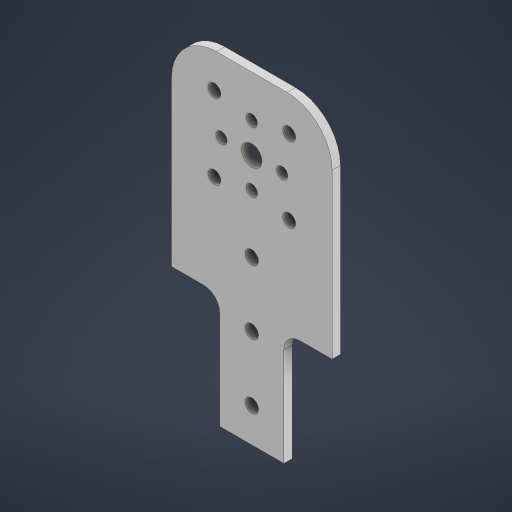
# Autodesk Inventor part: Arm Plate3
Saved by Autodesk Inventor 2024 (Build 280153000, 153)
## iProperties
Created: 2023-10-19
Part Number: Arm Plate3
Material: Generic
Document SubType Name: Modeling
Designer: ellen
Density: 1 g/cm^3
Appearance: Default
Author: ellen
Autodesk Inventor part; units mm, degrees
ref_plane "YZ Plane" through (0, 0, 0) normal (1, 0, 0) x (0, 1, 0)
ref_plane "XZ Plane" through (0, 0, 0) normal (0, 1, 0) x (-1, 0, 0)
ref_plane "XY Plane" through (0, 0, 0) normal (0, 0, 1) x (1, 0, 0)
sketch "Sketch1" plane through (0, 0, 0) normal (0, 0, 1) x (1, 0, 0)
  line L0 (63.5, 76.2) -> (0, 76.2)
  line L1 (0, 76.2) -> (0, 53.975)
  circle A0 centre (31.75, 47.625) radius 4.05
  line L2 (19.05, -6.35) -> (44.45, -6.35)
  line L3 (63.5, 53.975) -> (63.5, 76.2)
  line L4 (31.75, 76.2) -> (31.75, -6.35)
  circle A1 centre (31.75, 12.7) radius 2.6543
  circle A2 centre (31.75, -12.7) radius 2.6543
  circle A3 centre (31.75, -38.1) radius 2.6604
  line L5 (63.5, 53.975) -> (63.5, -6.35)
  line L6 (63.5, -6.35) -> (0, -6.35)
  line L7 (0, -6.35) -> (0, 53.975)
  line L8 (19.05, -6.35) -> (19.05, -51.598)
  line L9 (19.05, -51.598) -> (44.45, -51.598)
  line L10 (44.45, -51.598) -> (44.45, -6.35)
  point P0 (0, 0)
  dimension "d0" = 63.5
  dimension "d2" = 8.1
  dimension "d5" = 28.575
  dimension "d50" = 82.55
  dimension "d54" = 5.3086
  dimension "d55" = 63.5
  dimension "d59" = 25.4
  dimension "d60" = 25.4
  dimension "d61" = 25.4
  constraints: 22 end point, 5 perpendicular, 5 point on line, 4 centre point, 2 midpoint, 2 parallel, 2 vertical, 1 equal radius, 1 horizontal, 1 other
  measures "d0" distance of L0.end L0.start
  measures "d2" diameter of A0
  measures "d5" distance of A0.centre L4.start
  measures "d50" distance between parallel lines of L2 L0
  measures "d54" diameter of A1
  measures "d55" distance from line of L0 A1.centre
  measures "d59" distance of A2.centre A1.centre
  measures "d60" distance of A3.centre A2.centre
  measures "d61" distance of L8.end L9.end
extrude "Extrusion1" add sketch "Sketch1" along normal blind 3.302 contours L3 L5 L6 L2 L4 A1 A0 L0 | L4 A0 A1 L2 L6 L7 L1 L0 | L10 L9 L8 L2
fillet "Fillet11" radius 17.78 1 edges at (63.5, 76.2, 1.651)
fillet "Fillet12" radius 17.78 1 edges at (0, 76.2, 1.651)
sketch "Sketch3" plane through (0, 0, 3.302) normal (0, 0, 1) x (1, 0, 0)
  circle A0 centre (31.75, 47.625) radius 4.05 projected
  circle A1 centre (31.75, 47.625) radius 16
  circle A2 centre (31.75, 47.625) radius 8
  circle A3 centre (31.75, 47.625) radius 12
  line L0 (31.75, 47.625) -> (31.75, 69.8383)
  line L1 (31.75, 47.625) -> (53.9633, 47.625) construction
  point P0 (0, 0)
  point P1 (31.75, 59.625)
  dimension "d28" = 24
  dimension "d26" = 32
  dimension "d27" = 16
  dimension "d36" = 90
  constraints: 4 end point, 3 coincident, 2 centre point, 1 horizontal, 1 perpendicular, 1 point on line, 1 vertical alignment, 2 other
  measures "d26" diameter of A1
  measures "d27" diameter of A2
  measures "d36" angle of L1 L0
hole "Hole1" at (31.75, 59.625, 3.302) direction (0, 0, -1) diameter 4.4958 depth 14.1986 tip angle 118 clearance for "Flat Head Machine Screw" size "M4" standard "Ansi Metric M Profile"
pattern_circular "Circular Pattern1" count 4 over 360 about axis through (31.75, 47.625, 0) along (0, 0, 1) of "Hole1"
sketch "Sketch4" plane through (0, 0, 3.302) normal (0, 0, 1) x (1, 0, 0)
  circle A0 centre (31.75, 47.625) radius 4.05 projected
  circle A1 centre (31.75, 47.625) radius 12
  circle A2 centre (31.75, 47.625) radius 16
  circle A3 centre (31.75, 47.625) radius 20.955
  line L0 (45.72, 76.2) -> (17.78, 76.2) projected
  line L1 (31.75, 47.625) -> (51.1677, 67.0427)
  line L2 (31.75, 47.625) -> (59.2107, 47.625) construction
  point P0 (0, 0)
  point P1 (46.5674, 62.4424)
  dimension "d42" = 41.91
  dimension "d40" = 24
  dimension "d41" = 32
  dimension "d58" = 45
  constraints: 4 end point, 3 coincident, 2 centre point, 1 equal length, 1 horizontal, 1 point on line, 3 other
  measures "d40" diameter of A1
  measures "d41" diameter of A2
  measures "d58" angle of L2 L1
hole "Hole2" at (46.5674, 62.4424, 3.302) direction (0, 0, -1) diameter 5.1054 depth 16.256 tip angle 118 clearance for "Flat Head Machine Screw (82)" size "#10" standard "Ansi Unified Screw Threads"
pattern_circular "Circular Pattern2" count 4 over 360 about axis through (31.75, 47.625, 0) along (0, 0, 1) of "Hole2"
fillet "Fillet15" radius 6.35 2 edges at (44.45, -6.35, 1.651) (19.05, -6.35, 1.651)
equation "\"d54\" = d3"
equation "\"d3\" = 5.3086"
body "Solid1"
